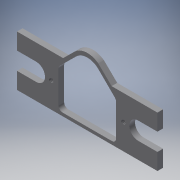
# Autodesk Inventor part: headplateLP_tapped
Saved by Autodesk Inventor 2016 (Build 200138000, 138)
## iProperties
Created: 2009-03-31
Part Number: headplateLP_tapped
Document SubType Name: Modeling
Designer: Daniel
Material: Generic
Density: 1 g/cm^3
Appearance: Default
Author: Daniel
Autodesk Inventor part; units mm, degrees
ref_plane "YZ Plane" through (0, 0, 0) normal (1, 0, 0) x (0, 1, 0)
ref_plane "XZ Plane" through (0, 0, 0) normal (0, 1, 0) x (-1, 0, 0)
ref_plane "XY Plane" through (0, 0, 0) normal (0, 0, 1) x (1, 0, 0)
sketch "Block1" plane through (0, 0, 0) normal (0, 0, 1) x (1, 0, 0)
  line L0 (-17.5911, -8.406) -> (-17.5911, -2.6569)
  arc A0 (-15.6308, 0.6431) -> (-17.4939, -2.2845) centre (9.5285, -17.4245) ccw
  arc A1 (-17.4939, -2.2845) -> (-17.5911, -2.6569) centre (-16.8291, -2.6569) ccw
  line L1 (-13.0521, -3.6322) -> (-2.9855, -3.6322)
  line L2 (-2.9855, -3.6322) -> (-2.9855, -10.0136)
  line L3 (-2.9855, -10.0136) -> (-13.0521, -10.0136)
  line L4 (-13.0521, -10.0136) -> (-13.0521, -3.6322)
  ellipse E0 centre (-8.0188, -3.6322) end of major axis (-8.0188, -7.4704) minor radius 2.9685
  point P0 (-13.9703, -5.5207)
  point P1 (-17.5911, -2.4593)
  dimension "d111" = 0.762
  measures "d111" radius of A1
sketch "Block2" plane through (0, 0, 0) normal (0, 0, 1) x (1, 0, 0)
  line L0 (-7.8958, -2.4967) -> (-7.8958, -8.4058)
  line L1 (-8.6339, -9.168) -> (-16.8291, -9.168)
  ellipse E0 centre (-12.6564, -2.1178) end of major axis (-12.6564, -6.4967) minor radius 3.853 (-9.6585, 0.6329) -> (-15.6415, 0.6509) ccw
  arc A0 (-7.8958, -2.4967) -> (-9.6091, 0.6391) centre (-35.8892, -15.7554) ccw
  line L2 (-17.6018, -8.3981) -> (-17.6018, -2.6491)
  arc A1 (-15.6415, 0.6509) -> (-17.5045, -2.2766) centre (9.5178, -17.4167) ccw
  arc A2 (-17.5045, -2.2766) -> (-17.6018, -2.6491) centre (-16.8398, -2.6491) ccw
  line L3 (-13.0627, -3.6243) -> (-2.9962, -3.6243)
  line L4 (-2.9962, -3.6243) -> (-2.9962, -10.0058)
  line L5 (-2.9962, -10.0058) -> (-13.0627, -10.0058)
  line L6 (-13.0627, -10.0058) -> (-13.0627, -3.6243)
  ellipse E1 centre (-8.0295, -3.6243) end of major axis (-8.0295, -7.4625) minor radius 2.9685
  point P0 (-12.2397, -5.1213)
sketch "Block3" plane through (0, 0, 0) normal (0, 0, 1) x (1, 0, 0)
  arc A0 (-17.5911, -8.406) -> (-16.8291, -9.168) centre (-16.8291, -8.406) ccw
  arc A1 (-8.6339, -9.168) -> (-7.8719, -8.406) centre (-8.6339, -8.406) ccw
  line L0 (-7.8958, -2.4967) -> (-7.8958, -8.4058)
  line L1 (-8.6339, -9.168) -> (-16.8291, -9.168)
  ellipse E0 centre (-12.6564, -2.1178) end of major axis (-12.6564, -6.4967) minor radius 3.853 (-9.6585, 0.6329) -> (-15.6415, 0.6509) ccw
  arc A2 (-7.8958, -2.4967) -> (-9.6091, 0.6391) centre (-35.8892, -15.7554) ccw
  line L2 (-17.6018, -8.3981) -> (-17.6018, -2.6491)
  arc A3 (-15.6415, 0.6509) -> (-17.5045, -2.2766) centre (9.5178, -17.4167) ccw
  arc A4 (-17.5045, -2.2766) -> (-17.6018, -2.6491) centre (-16.8398, -2.6491) ccw
  line L3 (-13.0627, -3.6243) -> (-2.9962, -3.6243)
  line L4 (-2.9962, -3.6243) -> (-2.9962, -10.0058)
  line L5 (-2.9962, -10.0058) -> (-13.0627, -10.0058)
  line L6 (-13.0627, -10.0058) -> (-13.0627, -3.6243)
  ellipse E1 centre (-8.0295, -3.6243) end of major axis (-8.0295, -7.4625) minor radius 2.9685
  point P0 (-12.6868, -8.3844)
  dimension "d110" = 0.762
  measures "d110" radius of A0
sketch "Block4" plane through (0, 0, 0) normal (0, 0, 1) x (1, 0, 0)
  arc A0 (-17.5911, -8.406) -> (-16.8291, -9.168) centre (-16.8291, -8.406) ccw
  arc A1 (-8.6339, -9.168) -> (-7.8719, -8.406) centre (-8.6339, -8.406) ccw
  line L0 (-7.8958, -2.4967) -> (-7.8958, -8.4058)
  line L1 (-8.6339, -9.168) -> (-16.8291, -9.168)
  ellipse E0 centre (-12.6564, -2.1178) end of major axis (-12.6564, -6.4967) minor radius 3.853 (-9.6585, 0.6329) -> (-15.6415, 0.6509) ccw
  arc A2 (-7.8958, -2.4967) -> (-9.6091, 0.6391) centre (-35.8892, -15.7554) ccw
  line L2 (-17.6018, -8.3981) -> (-17.6018, -2.6491)
  arc A3 (-15.6415, 0.6509) -> (-17.5045, -2.2766) centre (9.5178, -17.4167) ccw
  arc A4 (-17.5045, -2.2766) -> (-17.6018, -2.6491) centre (-16.8398, -2.6491) ccw
  line L3 (-13.0627, -3.6243) -> (-2.9962, -3.6243)
  line L4 (-2.9962, -3.6243) -> (-2.9962, -10.0058)
  line L5 (-2.9962, -10.0058) -> (-13.0627, -10.0058)
  line L6 (-13.0627, -10.0058) -> (-13.0627, -3.6243)
  ellipse E1 centre (-8.0295, -3.6243) end of major axis (-8.0295, -7.4625) minor radius 2.9685
  point P0 (-12.6868, -8.3844)
sketch "Block5" plane through (0, 0, 0) normal (0, 0, 1) x (1, 0, 0)
  ellipse E0 centre (-12.7876, -1.8459) end of major axis (-12.7876, -5.6516) minor radius 3.3457 (-10.6846, 1.114) -> (-14.8941, 1.1109) ccw
  arc A0 (-15.6984, 0.3796) -> (-14.8859, 1.1184) centre (-85.8065, 78.298) ccw
  arc A1 (-10.6894, 1.1184) -> (-9.8669, 0.3716) centre (60.1779, 78.3469) ccw
  point P0 (-12.7899, 8.9309)
sketch "Block6" plane through (0, 0, 0) normal (0, 0, 1) x (1, 0, 0)
  arc A0 (-10.9697, 1.4333) -> (-15.1792, 1.1122) centre (-12.8849, -1.2117) ccw
  line L0 (-15.1792, 1.1122) -> (-17.7718, -1.4473)
  line L1 (-10.8839, 1.361) -> (-8.0119, -1.4473)
  line L2 (-17.7718, -1.4473) -> (-8.0119, -1.4473)
  arc A1 (-10.8839, 1.361) -> (-10.9697, 1.4333) centre (-11.4166, 0.8161) ccw
  point P0 (-12.0633, -0.3449)
  point P1 (-10.9214, 1.3977)
  dimension "d153" = 0.762
  measures "d153" radius of A1
sketch "Sketch1" plane through (0, 0, 0) normal (0, 0, 1) x (1, 0, 0)
  line L0 (-25.4704, -0.3682) -> (-0.0704, -0.3682)
  line L1 (-0.0704, -0.3682) -> (-0.0704, -9.5122)
  line L2 (-0.0704, -9.5122) -> (-25.4704, -9.5122)
  line L3 (-25.4704, -9.5122) -> (-25.4704, -0.3682)
  constraints: 8 end point, 2 parallel, 1 horizontal, 1 perpendicular
extrude "Extrusion1" add sketch "Sketch1" along normal blind 1.016
sketch "Sketch2" plane through (0, 0, 1.016) normal (0, 0, 1) x (1, 0, 0)
  line L0 (-15.6279, -1.8922) -> (-9.9129, -1.8922)
  line L1 (-8.3254, -3.4797) -> (-8.3254, -6.4007)
  line L2 (-9.9129, -7.9882) -> (-15.6279, -7.9882)
  line L3 (-17.2154, -6.4007) -> (-17.2154, -3.4797)
  arc A0 (-15.6279, -1.8922) -> (-17.2154, -3.4797) centre (-15.6279, -3.4797) ccw
  arc A1 (-17.2154, -6.4007) -> (-15.6279, -7.9882) centre (-15.6279, -6.4007) ccw
  arc A2 (-9.9129, -7.9882) -> (-8.3254, -6.4007) centre (-9.9129, -6.4007) ccw
  arc A3 (-8.3254, -3.4797) -> (-9.9129, -1.8922) centre (-9.9129, -3.4797) ccw
  constraints: 8 end point, 8 point on circle, 8 tangent, 4 centre point, 3 equal radius, 2 parallel, 1 horizontal, 1 perpendicular
extrude "Extrusion2" cut sketch "Sketch2" against normal blind 1.016
sketch "Sketch3" plane through (0, 0, 1.016) normal (0, 0, 1) x (1, 0, 0)
  line L0 (-0.0704, -0.3682) -> (-0.0704, -9.5122) projected
  line L1 (-25.4704, -9.5122) -> (-25.4704, -0.3682) projected
  line L2 (-0.0704, -9.5122) -> (-25.4704, -9.5122) projected
  line L3 (-25.4704, -3.3527) -> (-21.9779, -3.3527)
  line L4 (-20.3904, -4.9402) -> (-20.3904, -4.9402)
  line L5 (-21.9779, -6.5277) -> (-25.4704, -6.5277)
  arc A0 (-20.3904, -4.9402) -> (-21.9779, -3.3527) centre (-21.9779, -4.9402) ccw
  arc A1 (-21.9779, -6.5277) -> (-20.3904, -4.9402) centre (-21.9779, -4.9402) ccw
  line L6 (-0.0704, -3.3527) -> (-3.5629, -3.3527)
  line L7 (-5.1504, -4.9402) -> (-5.1504, -4.9402)
  line L8 (-3.5629, -6.5277) -> (-0.0704, -6.5277)
  arc A2 (-3.5629, -3.3527) -> (-5.1504, -4.9402) centre (-3.5629, -4.9402) ccw
  arc A3 (-5.1504, -4.9402) -> (-3.5629, -6.5277) centre (-3.5629, -4.9402) ccw
  constraints: 12 end point, 8 point on circle, 8 tangent, 4 centre point, 4 perpendicular, 4 point on line, 2 concentric, 2 parallel
extrude "Extrusion3" cut sketch "Sketch3" against normal blind 1.016
sketch "Sketch13" plane through (0, 0, 1.016) normal (0, 0, 1) x (1, 0, 0)
  arc A0 (-10.8192, 2.023) -> (-15.0287, 1.7019) centre (-12.7344, -0.622) ccw
  line L0 (-15.0287, 1.7019) -> (-17.6213, -0.8576)
  line L1 (-10.7334, 1.9507) -> (-7.8614, -0.8576)
  line L2 (-17.6213, -0.8576) -> (-7.8614, -0.8576)
  arc A1 (-10.7334, 1.9507) -> (-10.8192, 2.023) centre (-11.2661, 1.4058) ccw
  point P0 (0, 0)
  point P1 (0, 0)
  point P2 (0, 0)
extrude "Extrusion8" add sketch "Sketch13" against normal blind 1.016
sketch "Sketch12" plane through (0, 0, 1.016) normal (0, 0, 1) x (1, 0, 0)
  line L0 (-7.5424, -2.4012) -> (-7.5424, -8.1771)
  line L1 (-8.3044, -8.9391) -> (-17.2004, -8.9391)
  line L2 (-17.9624, -2.4) -> (-17.9624, -8.1771)
  arc A0 (-17.9624, -8.1771) -> (-17.2004, -8.9391) centre (-17.2004, -8.1771) ccw
  arc A1 (-8.3044, -8.9391) -> (-7.5424, -8.1771) centre (-8.3044, -8.1771) ccw
  line L3 (-10.8562, 1.2031) -> (-7.7678, -1.8602)
  line L4 (-14.7403, 1.0994) -> (-17.7357, -1.8577)
  arc A2 (-10.847, 1.1949) -> (-14.7403, 1.0994) centre (-12.7429, -0.9239) ccw
  arc A3 (-17.7357, -1.8577) -> (-17.9624, -2.4) centre (-17.2004, -2.4) ccw
  arc A4 (-7.5424, -2.4012) -> (-7.7678, -1.8602) centre (-8.3044, -2.4012) ccw
  point P0 (0, 0)
  point P1 (-17.1532, -8.9391)
  point P2 (-17.9624, -7.9131)
  point P3 (-7.5424, -8.1803)
  point P4 (-8.3956, -8.9391)
  point P5 (0, 0)
  point P6 (-17.6124, -1.736)
  point P7 (-17.9624, -2.2782)
  point P8 (-7.8931, -1.7359)
  point P9 (-7.5424, -2.2782)
  dimension "d149" = 0.762
  dimension "d150" = 0.762
  dimension "d154" = 0.762
  constraints: 11 point on circle, 10 end point, 9 tangent, 8 point on line, 5 centre point, 2 vertical, 1 equal radius
  measures "d149" radius of A0
  measures "d150" radius of A1
  measures "d154" radius of A3
extrude "Extrusion7" cut sketch "Sketch12" against normal blind 1.016
hole "Hole9" at (-19.2355, -4.93, 1.016) direction (0, 0, -1) diameter 0.7366 depth 1.524
hole "Hole10" at (-6.1975, -4.9172, 1.016) direction (0, 0, -1) diameter 0.7366 depth 2.794
body "Solid1"
